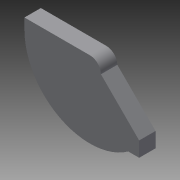
# Autodesk Inventor part: nd-gate
Saved by Autodesk Inventor 2015 (Build 190159000, 159)
## iProperties
Created: 2014-07-02
Part Number: nd-gate
Material: Generic
Document SubType Name: Modeling
Designer: peter
Density: 1 g/cm^3
Appearance: Default
Author: peter
Autodesk Inventor part; units mm, degrees
ref_plane "YZ Plane" through (0, 0, 0) normal (1, 0, 0) x (0, 1, 0)
ref_plane "XZ Plane" through (0, 0, 0) normal (0, 1, 0) x (-1, 0, 0)
ref_plane "XY Plane" through (0, 0, 0) normal (0, 0, 1) x (1, 0, 0)
sketch "Sketch1" plane through (0, 0, 0) normal (0, 0, 1) x (1, 0, 0)
  arc A0 (0.0426, 76.2427) -> (120.6926, 14.3506) centre (76.2426, 76.2427) ccw
  line L0 (0.0426, 88.9427) -> (0.0426, 76.2427)
  line L1 (76.2426, 88.9427) -> (0.0426, 88.9427)
  arc A1 (88.9426, 76.2427) -> (76.2426, 88.9427) centre (76.2426, 76.2427) ccw
  line L2 (133.3926, 31.7927) -> (88.9426, 76.2427)
  line L3 (120.6926, 14.3506) -> (133.3926, 14.3506)
  line L4 (133.3926, 14.3506) -> (133.3926, 31.7927)
  point P0 (0, 0)
  constraints: 10 end point, 4 point on circle, 2 centre point
extrude "Extrusion1" add sketch "Sketch1" along normal blind 19.05
body "Solid1"
